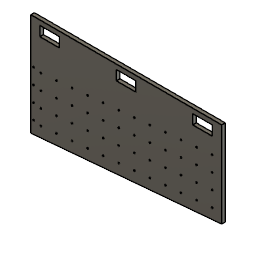
_ShelfBoard.81033265-85c9-4357-85a3-4fb4a8ea5411 (Autodesk Fusion 360 design; units mm, degrees)
Autodesk Fusion 360 part; units mm, degrees
note: some values were not read from the file. Set by a fixed rule: which sketch regions a step uses.
sketch "Sketch1" plane through (0, 0, 0) normal (0, 0, 1) x (1, 0, 0)
  line L0 (0, 0) -> (-1000, 0)
  line L1 (0, 0) -> (0, -450)
  line L2 (0, -450) -> (-1000, -537.4887)
  line L3 (-1000, 0) -> (-1000, -537.4887)
  dimension "d4" = 95
  constraint coincident L0.start L1.start
  constraint horizontal L0
  constraint perpendicular L0 L1
  constraint perpendicular L0 L3
  measures "d4" angle of L1 L2
extrude "Extrude1" add sketch "Sketch1" along normal blind 19.05
sketch "Sketch2" plane through (0, 0, 19.05) normal (0, 0, 1) x (1, 0, 0)
  line L0 (0, 0) -> (-1000, 0)
  line L1 (-1000, 0) -> (-1000, -537.4887)
  line L2 (-1000, -537.4887) -> (0, -450)
  line L3 (0, -450) -> (0, 0)
  circle A0 centre (-50, -400) radius 4
  circle A1 centre (-149.6066, 738.5082) radius 4
  circle A2 centre (-277.6887, 727.3025) radius 4
  circle A3 centre (-405.7709, 716.0967) radius 4
  circle A4 centre (-533.8531, 704.891) radius 4
  circle A5 centre (-661.9353, 693.6853) radius 4
  circle A6 centre (-790.0174, 682.4795) radius 4
  circle A7 centre (-918.0996, 671.2738) radius 4
  circle A8 centre (-1046.1818, 660.0681) radius 4
  circle A9 centre (-249.2131, 1877.0165) radius 4
  circle A10 centre (-377.2953, 1865.8107) radius 4
  circle A11 centre (-505.3775, 1854.605) radius 4
  circle A12 centre (-633.4597, 1843.3992) radius 4
  circle A13 centre (-761.5418, 1832.1935) radius 4
  circle A14 centre (-889.624, 1820.9878) radius 4
  circle A15 centre (-1017.7062, 1809.782) radius 4
  circle A16 centre (-1145.7884, 1798.5763) radius 4
  circle A17 centre (-348.8197, 3015.5247) radius 4
  circle A18 centre (-476.9019, 3004.3189) radius 4
  circle A19 centre (-604.984, 2993.1132) radius 4
  circle A20 centre (-733.0662, 2981.9075) radius 4
  circle A21 centre (-861.1484, 2970.7017) radius 4
  circle A22 centre (-989.2306, 2959.496) radius 4
  circle A23 centre (-1117.3127, 2948.2902) radius 4
  circle A24 centre (-1245.3949, 2937.0845) radius 4
  circle A25 centre (-448.4263, 4154.0329) radius 4
  circle A26 centre (-576.5084, 4142.8272) radius 4
  circle A27 centre (-704.5906, 4131.6214) radius 4
  circle A28 centre (-832.6728, 4120.4157) radius 4
  circle A29 centre (-960.755, 4109.21) radius 4
  circle A30 centre (-1088.8371, 4098.0042) radius 4
  circle A31 centre (-1216.9193, 4086.7985) radius 4
  circle A32 centre (-1345.0015, 4075.5927) radius 4
  circle A33 centre (-548.0328, 5292.5411) radius 4
  circle A34 centre (-676.115, 5281.3354) radius 4
  circle A35 centre (-804.1972, 5270.1297) radius 4
  circle A36 centre (-932.2793, 5258.9239) radius 4
  circle A37 centre (-1060.3615, 5247.7182) radius 4
  circle A38 centre (-1188.4437, 5236.5124) radius 4
  circle A39 centre (-1316.5259, 5225.3067) radius 4
  circle A40 centre (-1444.608, 5214.101) radius 4
  circle A41 centre (-647.6394, 6431.0494) radius 4
  circle A42 centre (-775.7216, 6419.8436) radius 4
  circle A43 centre (-903.8037, 6408.6379) radius 4
  circle A44 centre (-1031.8859, 6397.4321) radius 4
  circle A45 centre (-1159.9681, 6386.2264) radius 4
  circle A46 centre (-1288.0503, 6375.0207) radius 4
  circle A47 centre (-1416.1324, 6363.8149) radius 4
  circle A48 centre (-1544.2146, 6352.6092) radius 4
  circle A49 centre (-747.2459, 7569.5576) radius 4
  circle A50 centre (-875.3281, 7558.3518) radius 4
  circle A51 centre (-1003.4103, 7547.1461) radius 4
  circle A52 centre (-1131.4925, 7535.9404) radius 4
  circle A53 centre (-1259.5746, 7524.7346) radius 4
  circle A54 centre (-1387.6568, 7513.5289) radius 4
  circle A55 centre (-1515.739, 7502.3232) radius 4
  circle A56 centre (-1643.8212, 7491.1174) radius 4
extrude "Extrude2" cut sketch "Sketch2" against normal blind 250 contours A0
pattern_linear "R-Pattern1" count 12 spacing 81.8182 along (-0.996195, -0.087156, 0) of "Extrude2"
pattern_linear "R-Pattern2" count 4 spacing 80 along (0, 1, 0) of "Extrude2", "R-Pattern1"
sketch "Sketch3" plane through (0, 0, 19.05) normal (0, 0, 1) x (1, 0, 0)
  circle A0 centre (-946.5752, -238.4402) radius 4
  circle A1 centre (-865.0684, -231.3092) radius 4
  circle A2 centre (-783.5616, -224.1783) radius 4
  circle A3 centre (-702.0547, -217.0474) radius 4
  circle A4 centre (-620.5479, -209.9165) radius 4
  circle A5 centre (-539.041, -202.7855) radius 4
  circle A6 centre (-457.5342, -195.6546) radius 4
  circle A7 centre (-376.0274, -188.5237) radius 4
  circle A8 centre (-294.5205, -181.3928) radius 4
  circle A9 centre (-213.0137, -174.2618) radius 4
  circle A10 centre (-131.5068, -167.1309) radius 4
  circle A11 centre (-50, -160) radius 4
  circle A12 centre (-946.5752, -318.4402) radius 4
  circle A13 centre (-865.0684, -311.3092) radius 4
  circle A14 centre (-783.5616, -304.1783) radius 4
  circle A15 centre (-702.0547, -297.0474) radius 4
  circle A16 centre (-620.5479, -289.9165) radius 4
  circle A17 centre (-539.041, -282.7855) radius 4
  circle A18 centre (-457.5342, -275.6546) radius 4
  circle A19 centre (-376.0274, -268.5237) radius 4
  circle A20 centre (-294.5205, -261.3928) radius 4
  circle A21 centre (-213.0137, -254.2618) radius 4
  circle A22 centre (-131.5068, -247.1309) radius 4
  circle A23 centre (-50, -240) radius 4
  circle A24 centre (-946.5752, -398.4402) radius 4
  circle A25 centre (-865.0684, -391.3092) radius 4
  circle A26 centre (-783.5616, -384.1783) radius 4
  circle A27 centre (-702.0547, -377.0474) radius 4
  circle A28 centre (-620.5479, -369.9165) radius 4
  circle A29 centre (-539.041, -362.7855) radius 4
  circle A30 centre (-457.5342, -355.6546) radius 4
  circle A31 centre (-376.0274, -348.5237) radius 4
  circle A32 centre (-294.5205, -341.3928) radius 4
  circle A33 centre (-213.0137, -334.2618) radius 4
  circle A34 centre (-131.5068, -327.1309) radius 4
  circle A35 centre (-50, -320) radius 4
  circle A36 centre (-946.5752, -478.4402) radius 4
  circle A37 centre (-865.0684, -471.3092) radius 4
  circle A38 centre (-783.5616, -464.1783) radius 4
  circle A39 centre (-702.0547, -457.0474) radius 4
  circle A40 centre (-620.5479, -449.9165) radius 4
  circle A41 centre (-539.041, -442.7855) radius 4
  circle A42 centre (-457.5342, -435.6546) radius 4
  circle A43 centre (-376.0274, -428.5237) radius 4
  circle A44 centre (-294.5205, -421.3928) radius 4
  circle A45 centre (-213.0137, -414.2618) radius 4
  circle A46 centre (-131.5068, -407.1309) radius 4
  circle A47 centre (-50, -400) radius 4
  line L0 (0, 0) -> (-1000, 0)
  line L1 (-1000, 0) -> (-1000, -537.4887)
  line L2 (-1000, -537.4887) -> (0, -450)
  line L3 (0, -450) -> (0, 0)
  line L4 (-151.6, -25) -> (-50, -25)
  line L5 (-50, -25) -> (-50, -75.8)
  line L6 (-50, -75.8) -> (-151.6, -75.8)
  line L7 (-151.6, -75.8) -> (-151.6, -25)
  constraint horizontal L4
  constraint vertical L5
  constraint horizontal L6
  constraint vertical L7
extrude "Extrude3" cut sketch "Sketch3" against normal blind 160 contours L4 L5 L6 L7
pattern_linear "R-Pattern3" count 3 spacing 400 along (-1, 0, 0) of "Extrude3"
sketch "Sketch4" plane through (0, 0, 19.05) normal (0, 0, 1) x (1, 0, 0)
  line L0 (-850, -25) -> (-850, -75.8)
  line L1 (-850, -75.8) -> (-951.6, -75.8)
  line L2 (-951.6, -75.8) -> (-951.6, -25)
  line L3 (-951.6, -25) -> (-850, -25)
  line L4 (-450, -25) -> (-450, -75.8)
  line L5 (-450, -75.8) -> (-551.6, -75.8)
  line L6 (-551.6, -75.8) -> (-551.6, -25)
  line L7 (-551.6, -25) -> (-450, -25)
  line L8 (-50, -25) -> (-50, -75.8)
  line L9 (-50, -75.8) -> (-151.6, -75.8)
  line L10 (-151.6, -75.8) -> (-151.6, -25)
  line L11 (-151.6, -25) -> (-50, -25)
  circle A0 centre (-946.5752, -238.4402) radius 4
  circle A1 centre (-865.0684, -231.3092) radius 4
  circle A2 centre (-783.5616, -224.1783) radius 4
  circle A3 centre (-702.0547, -217.0474) radius 4
  circle A4 centre (-620.5479, -209.9165) radius 4
  circle A5 centre (-539.041, -202.7855) radius 4
  circle A6 centre (-457.5342, -195.6546) radius 4
  circle A7 centre (-376.0274, -188.5237) radius 4
  circle A8 centre (-294.5205, -181.3928) radius 4
  circle A9 centre (-213.0137, -174.2618) radius 4
  circle A10 centre (-131.5068, -167.1309) radius 4
  circle A11 centre (-50, -160) radius 4
  circle A12 centre (-946.5752, -318.4402) radius 4
  circle A13 centre (-865.0684, -311.3092) radius 4
  circle A14 centre (-783.5616, -304.1783) radius 4
  circle A15 centre (-702.0547, -297.0474) radius 4
  circle A16 centre (-620.5479, -289.9165) radius 4
  circle A17 centre (-539.041, -282.7855) radius 4
  circle A18 centre (-457.5342, -275.6546) radius 4
  circle A19 centre (-376.0274, -268.5237) radius 4
  circle A20 centre (-294.5205, -261.3928) radius 4
  circle A21 centre (-213.0137, -254.2618) radius 4
  circle A22 centre (-131.5068, -247.1309) radius 4
  circle A23 centre (-50, -240) radius 4
  circle A24 centre (-946.5752, -398.4402) radius 4
  circle A25 centre (-865.0684, -391.3092) radius 4
  circle A26 centre (-783.5616, -384.1783) radius 4
  circle A27 centre (-702.0547, -377.0474) radius 4
  circle A28 centre (-620.5479, -369.9165) radius 4
  circle A29 centre (-539.041, -362.7855) radius 4
  circle A30 centre (-457.5342, -355.6546) radius 4
  circle A31 centre (-376.0274, -348.5237) radius 4
  circle A32 centre (-294.5205, -341.3928) radius 4
  circle A33 centre (-213.0137, -334.2618) radius 4
  circle A34 centre (-131.5068, -327.1309) radius 4
  circle A35 centre (-50, -320) radius 4
  circle A36 centre (-946.5752, -478.4402) radius 4
  circle A37 centre (-865.0684, -471.3092) radius 4
  circle A38 centre (-783.5616, -464.1783) radius 4
  circle A39 centre (-702.0547, -457.0474) radius 4
  circle A40 centre (-620.5479, -449.9165) radius 4
  circle A41 centre (-539.041, -442.7855) radius 4
  circle A42 centre (-457.5342, -435.6546) radius 4
  circle A43 centre (-376.0274, -428.5237) radius 4
  circle A44 centre (-294.5205, -421.3928) radius 4
  circle A45 centre (-213.0137, -414.2618) radius 4
  circle A46 centre (-131.5068, -407.1309) radius 4
  circle A47 centre (-50, -400) radius 4
  line L12 (0, 0) -> (-1000, 0)
  line L13 (-1000, 0) -> (-1000, -537.4887)
  line L14 (-1000, -537.4887) -> (0, -450)
  line L15 (0, -450) -> (0, 0)
  line L16 (-946.5752, -478.4402) -> (-865.0684, -471.3092)
  line L17 (-946.9239, -474.4554) -> (-865.417, -467.3245)
  circle A48 centre (-946.5752, -478.4402) radius 11
  line L18 (-1000, -472.0722) -> (-1000, -477.3421)
  circle A49 centre (-985.3453, -471.4402) radius 4
  line L19 (-981.9143, -473.4964) -> (-983.6579, -472.462)
  line L20 (-975, -469.885) -> (-938.2096, -466.6663)
  constraint coincident A36.centre L16.start
  constraint coincident A37.centre L16.end
  constraint coincident L13 L18.end
  constraint coincident A49 L19.start
extrude "Extrude4" cut sketch "Sketch4" against normal blind 40 contours A49
pattern_linear "R-Pattern4" count 4 spacing 80 along (0, 1, 0) of "Extrude4"
